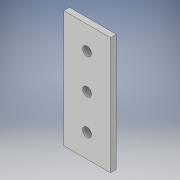
# Autodesk Inventor part: CLB_040_ScissorLiftSpacer
Saved by Autodesk Inventor 2018.3 (Build 223284000, 284)
## iProperties
Created: 2020-01-31
Part Number: CLB_040_ScissorLiftSpacer
Material: Generic
Document SubType Name: Modeling
Designer: Cooper
Density: 1 g/cm^3
Appearance: Default
Author: Cooper
Autodesk Inventor part; units mm, degrees
ref_plane "YZ Plane" through (0, 0, 0) normal (1, 0, 0) x (0, 1, 0)
ref_plane "XZ Plane" through (0, 0, 0) normal (0, 1, 0) x (-1, 0, 0)
ref_plane "XY Plane" through (0, 0, 0) normal (0, 0, 1) x (1, 0, 0)
sketch "Sketch1" plane through (0, 0, 0) normal (0, 0, 1) x (1, 0, 0)
  line L0 (0, 0) -> (25.4, 0)
  line L1 (25.4, 0) -> (25.4, 63.5)
  line L2 (25.4, 63.5) -> (0, 63.5)
  line L3 (0, 63.5) -> (0, 0)
  dimension "d0" = 25.4
  dimension "d1" = 63.5
  constraints: 8 end point, 2 parallel, 1 horizontal, 1 perpendicular
  measures "d0" distance of L0.start L0.end
  measures "d1" distance of L2.end L0.start
extrude "Extrusion1" add sketch "Sketch1" along normal blind 3.175
sketch "Sketch2" plane through (0, 0, 3.175) normal (0, 0, 1) x (1, 0, 0)
  line L0 (0, 0) -> (25.4, 0) projected
  line L1 (25.4, 0) -> (25.4, 63.5) projected
  line L2 (25.4, 63.5) -> (0, 63.5) projected
  line L3 (0, 63.5) -> (0, 0) projected
  point P0 (12.7, 12.7)
  point P1 (12.7, 50.8)
  point P2 (12.7, 31.75)
  dimension "d4" = 12.7
  dimension "d5" = 12.7
  dimension "d6" = 12.7
  dimension "d18" = 19.05
  dimension "d19" = 19.05
  constraints: 2 vertical alignment
  measures "d4" distance from line of L3 point (12.7, 12.7)
  measures "d5" distance from line of L1 point (12.7, 12.7)
  measures "d6" distance from line of L0 point (12.7, 12.7)
  measures "d18" distance of point (12.7, 12.7) point (12.7, 31.75)
  measures "d19" distance of point (12.7, 50.8) point (12.7, 31.75)
hole "Hole1" at (12.7, 12.7, 3.175) at (12.7, 31.75, 3.175) at (12.7, 50.8, 3.175) direction (0, 0, -1) diameter 4.8514 end through all
equation "\"d4\" = d5"
body "Solid1"
